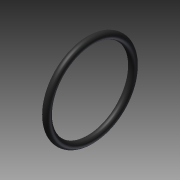
# Autodesk Inventor part: 9452K87 Buna-N O-Ring
Saved by Autodesk Inventor 2012 SP1 (Build 160190100, 190)
## iProperties
Created: 2012-06-04
Part Number: 9452K87 Buna-N O-Ring
Material: Rubber
Document SubType Name: Modeling
Designer: ding42
Mass: 0.506575 g
Surface Area: 8.35005 cm^2
Volume: 0.544705 cm^3
Density: 0.93 g/cm^3
Description: Dash Number 123
Author: ding42
Autodesk Inventor part; units mm, degrees
ref_plane "YZ Plane" through (0, 0, 0) normal (1, 0, 0) x (0, 1, 0)
ref_plane "XZ Plane" through (0, 0, 0) normal (0, 1, 0) x (-1, 0, 0)
ref_plane "XY Plane" through (0, 0, 0) normal (0, 0, 1) x (1, 0, 0)
sketch "Sketch1" plane through (0, 0, 0) normal (0, 0, 1) x (1, 0, 0)
  circle A0 centre (0, 0) radius 1.3081
  dimension "d0" = 2.6162
  constraints: 1 centre point, 1 coincident
  measures "d0" diameter of A0
sketch "Sketch2" plane through (0, 0, 0) normal (1, 0, 0) x (0, 1, 0)
  circle A0 centre (16.1269, -1.645) radius 14.9098
  line L0 (1.3081, 0) -> (-1.3081, 0) projected
  point P0 (0, 0)
  dimension "d1" = 29.8196
  constraints: 3 other
sweep "Sweep1" add profiles "Sketch1" path "Sketch2" path curves A0
body "Solid1"
